encoder wheel_v3 (Autodesk Fusion 360 design; units mm, degrees)
Autodesk Fusion 360 part; units mm, degrees
sketch "Sketch1" plane through (0, 0, 0) normal (0, 1, 0) x (1, 0, 0) in component "hub"
  circle A0 centre (0, 0) radius 28
  circle A1 centre (0, 0) radius 13
  circle A2 centre (0, 0) radius 2
  dimension "d1" = 56
  dimension "d2" = 26
  dimension "d3" = 4
  constraint coincident A0.centre A1.centre
  constraint concentric A0 A1
  measures "d1" diameter of A0
  measures "d2" diameter of A1
  measures "d3" diameter of A2
extrude "Extrude1" add sketch "Sketch1" against normal blind 6 contours A0 | A1 | A2 makes body 1 in component "hub"
extrude "Extrude2" add sketch "Sketch1" along normal blind 5.5 contours A1 bodies 1 in component "hub"
extrude "Extrude3" cut 1 faces at (0.637, 0, -0.1965) along direction (0, -1, 0) through all on bodies 1 bodies 1 in component "hub"
sketch "Sketch2" plane through (0, 0, 0) normal (1, 0, 0) x (0, -1, 0) in component "hub"
  line L0 (6, -28) -> (6, 28) construction
  line L1 (0, 28) -> (0, -28) construction
  line L2 (6, -28) -> (5.5, -28) construction
  line L3 (0, -28) -> (0.5, -28) construction
  line L4 (5.5, -28) -> (0.5, -28) construction
  line L5 (3, -28) -> (3, -26.5) construction
  circle A0 centre (3, -29.3333) radius 2.8333
  dimension "d8" = 0.5
  dimension "d9" = 0.5
  dimension "d10" = 1.5
  constraint coincident L0.start L2.start
  constraint perpendicular L0 L2
  constraint coincident L1.end L3.start
  constraint perpendicular L1 L3
  constraint midpoint L4 L5.start
  constraint perpendicular L4 L5
  constraint coincident L2.end A0
  constraint coincident L5.end A0
  constraint coincident L3.end A0
  measures "d8" distance of L0.start L2.end
  measures "d9" distance of L1.end L3.end
  measures "d10" distance of L5.start L5.end
revolve "Revolve1" cut sketch "Sketch2" angle 360 about axis through (0, 1.75, 0) along (0, 1, 0) bodies 1 in component "hub"
sketch "Sketch1 (2)" plane through (0, 0, 0) normal (1, 0, 0) x (0, 1, 0) in component "wheel"
  circle A0 centre (-3, 29.3333) radius 2.8333
revolve "Revolve1'" add sketch "Sketch1 (2)" angle 360 about axis through (0, 1.75, 0) along (0, 1, 0) separate body makes body 2 in component "wheel"
component "hub" placed x (1, 0, 0) y (0, 1, 0) z (0, 0, 1) at (0, 0, 0)
component "wheel" placed x (1, 0, 0) y (0, 1, 0) z (0, 0, 1) at (0, 0, 0)
